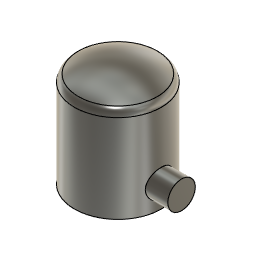
STack_Holder v3 (Autodesk Fusion 360 archive; units mm, degrees)
design "PAr"
Autodesk Fusion 360 part; units mm, degrees
sketch "Sketch1" plane through (0, 0, 0) normal (1, 0, 0) x (0, 1, 0)
  line L0 (0, 0) -> (0, 87.265)
  line L1 (-15, 0) -> (-15, 32)
  circle A0 centre (0, 12) radius 25
  line L2 (-15, 0) -> (0, 0)
  point P0 (0, 37)
  dimension "d2" = 30
  dimension "d3" = 12
  dimension "d4" = 37
  constraint coincident L0.start L2.end
  constraint vertical L0
  constraint vertical L1
  constraint coincident L0 A0.centre
  constraint coincident L1.end A0
  constraint horizontal L2
  constraint coincident L0 P0
  constraint coincident A0 P0
  measures "d3" distance of L0.start A0.centre
  measures "d4" distance of L0.start P0
revolve "Revolve1" add sketch "Sketch1" angle 360 about axis through (0, 0, 0) along (0, 0, 1) contours L0 L1 A0 L2 picked at (-10, 10.6667)
fillet "Fillet1" radius 3 1 edges at (-13.9849, -5.4242, 32)
sketch "Sketch2" plane through (0, 0, 0) normal (1, 0, 0) x (0, 1, 0)
  circle A0 centre (0, 7.75) radius 4.75
  line L0 (0, 0) -> (0, 38.3314) construction
  dimension "d8" = 9.5
  dimension "d9" = 7.75
  constraint coincident L0.start origin
  constraint vertical L0
  constraint coincident A0.centre L0
  measures "d8" diameter of A0
  measures "d9" distance of L0.start A0.centre
extrude "Extrude1" add sketch "Sketch2" along normal blind 22
sketch "Sketch3" plane through (0, 0, 0) normal (0, 0, -1) x (1, 0, 0)
  circle A0 centre (0, 0) radius 15
  line L0 (0, 0) -> (-12.5, 0) construction
  circle A1 centre (-12.5, 0) radius 2
  line L1 (15, 0) -> (15, -13) construction
  dimension "d12" = 4
  dimension "d13" = 27.5
  constraint coincident A0.centre L0.start
  constraint horizontal L0
  constraint coincident L0.end A1.centre
  constraint coincident A0 L1.start
  constraint tangent A0 L1
  constraint perpendicular L0 L1
  measures "d12" diameter of A1
  measures "d13" distance of L0.end L1
extrude "Extrude2" cut sketch "Sketch3" against normal blind 8 contours A1
equation "d9 = 12.5 mm - d8 / 2"
equation "d10 = 37 mm - ( 30 / 2 ) * 1 mm"
equation "d13 = 25.5 mm + d12 / 2"

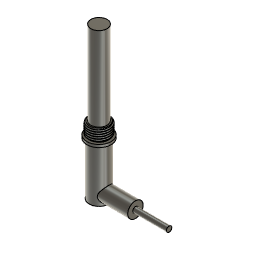
design "EE-08-SS"
Autodesk Fusion 360 part; units mm, degrees
sketch "Sketch1" plane through (0, 0, 0) normal (1, 0, 0) x (0, 1, 0) in component "EE-08-M1A8"
  line L0 (0, 0) -> (0, 115)
  line L1 (0, 0) -> (-6, 0)
  line L2 (-6, 0) -> (-6, 12)
  line L3 (-6, 12) -> (-9, 12)
  line L4 (-9, 12) -> (-9, 14)
  line L5 (-9, 14) -> (-8, 14)
  line L6 (-8, 14) -> (-8, 23)
  line L7 (-8, 23) -> (-6, 23)
  line L8 (-6, 23) -> (-6, 85)
  line L9 (-6, 85) -> (0, 85)
  line L10 (-8, 14) -> (-7, 14)
  line L11 (-7, 14) -> (-8, 15)
  line L12 (-7, 23) -> (-8, 22)
  dimension "d2" = 12
  dimension "d3" = 12
  dimension "d4" = 18
  dimension "d5" = 2
  dimension "d6" = 9
  dimension "d7" = 16
  dimension "d8" = 12
  dimension "d9" = 71
  dimension "d12" = 14
  dimension "d13" = 45
  dimension "d15" = 14
  constraint coincident L0.start L1.start
  constraint vertical L0
  constraint perpendicular L0 L1
  constraint perpendicular L1 L2
  constraint perpendicular L2 L3
  constraint perpendicular L3 L4
  constraint perpendicular L0 L5
  constraint perpendicular L5 L6
  constraint perpendicular L6 L7
  constraint perpendicular L5 L8
  constraint coincident L0 L9.end
  constraint perpendicular L0 L9
  constraint perpendicular L6 L10
  constraint coincident L6 L11.end
  constraint coincident L6 L12.end
  constraint perpendicular L11 L12
  constraint coincident L7 L12.start
  measures "d3" distance of L1.end L2.end
  measures "d5" distance of L3 L5.end
  measures "d6" distance of L5.end L6.end
  measures "d9" distance of L4.end L9
  measures "d13" angle of L7 L12
revolve "Revolve1" add sketch "Sketch1" angle 360 about axis through (0, 0, 0) along (0, 0, 1) makes body 1
thread "Thread1" "ISO Metric profile 16.0 M16x1.5 6g" major diameter 15.85 minor diameter 14.137 pitch 1.5 angle 60 modelled right hand crest width 0.2154 on face at (-0.3988, -7.9901, 22.3333) crest through (0, -7.925, 13.625) on face at (-0.7965, -7.9602, 19.6667) crest through (0, -7.925, 13.625) on face at (-0.7965, -7.9602, 14.3333) crest through (0, -7.925, 13.625) on bodies 1
revolve "Revolve2" cut sketch "Sketch1" angle 360 about axis through (0, 0, 0) along (0, 0, 1) contours L6 L7 L12 | L6 L10 L11 bodies 1
sketch "Sketch1 (2)" plane through (0, 0, 0) normal (1, 0, 0) x (0, 1, 0)
  line L0 (0, 0) -> (0, 25)
  line L1 (-9.7, 25.5) -> (-6.75, 25.5)
  line L2 (-6.75, 25.5) -> (-6.75, 14)
  line L3 (-6.75, 14) -> (-9.7, 14)
  line L4 (-9.7, 14) -> (-9.7, 25.5)
  line L5 (6.75, 25.5) -> (10.5012, 25.5)
  line L6 (10.5012, 25.5) -> (10.5012, 14)
  line L7 (10.5012, 14) -> (6.75, 14)
  line L8 (6.75, 14) -> (6.75, 25.5)
  line L9 (0, 0) -> (0, 115)
  dimension "d17" = 6.75
  dimension "d18" = 6.75
  constraint vertical L0
  constraint coincident L0.start L9.start
  constraint horizontal L1
  constraint vertical L2
  constraint horizontal L3
  constraint vertical L4
  constraint horizontal L5
  constraint vertical L6
  constraint horizontal L7
  constraint vertical L8
  measures "d17" distance of L8 L9
  measures "d18" distance of L0.end L2
sketch "Sketch2" plane through (0, 0, 0) normal (0, 1, 0) x (1, 0, 0)
sketch "Sketch1 (3)" plane through (0, 0, 12) normal (0, 0, -1) x (1, 0, 0) in component "wire"
  circle A0 centre (0, 0) radius 6
  circle A1 centre (0, 0) radius 9
  circle A2 centre (0, 0) radius 7.25
  dimension "d21" = 14.5
  constraint concentric A0 A2
  measures "d21" diameter of A2
extrude "Extrude1" add sketch "Sketch1 (3)" along normal blind 39 separate body contours A0 | A2 makes body 2 in component "wire"
sketch "Sketch2 (2)" plane through (0, 0, 0) normal (1, 0, 0) x (0, 1, 0) in component "wire"
  circle A0 centre (0, -20.7) radius 5.7
  line L0 (9, 12) -> (-9, 12)
  line L1 (0, 12) -> (0, -36) construction
  dimension "d24" = 11.4
  dimension "d25" = 32.7
  constraint midpoint L0 L1.start
  constraint perpendicular L0 L1
  constraint coincident A0.centre L1
  measures "d24" diameter of A0
  measures "d25" distance of A0.centre L0
extrude "Extrude2" add sketch "Sketch2 (2)" along normal blind 27 bodies 2 in component "wire"
sketch "Sketch3" plane through (27, 0, 0) normal (1, 0, 0) x (0, 1, 0) in component "wire"
  circle A0 centre (0, -20.7) radius 5.7
  circle A1 centre (0, -20.7) radius 2
  dimension "d28" = 4
  constraint concentric A0 A1
  measures "d28" diameter of A1
extrude "Extrude3" add sketch "Sketch3" along normal blind 25 contours A1 bodies 2 in component "wire"
extrude "Extrude1'" [rolled back] along distance 16.5 taper angle 0
component "EE-08-M1A8" placed x (1, 0, 0) y (0, 1, 0) z (0, 0, 1) at (0, 0, 0)
component "wire" placed x (1, 0, 0) y (0, 1, 0) z (0, 0, 1) at (0, 0, 0)
equation "d15 = d12"
equation "d17 = ( 13.5 / 2 ) * 1 mm"
equation "d18 = d17"
equation "d25 = 27 mm + d24 / 2"
